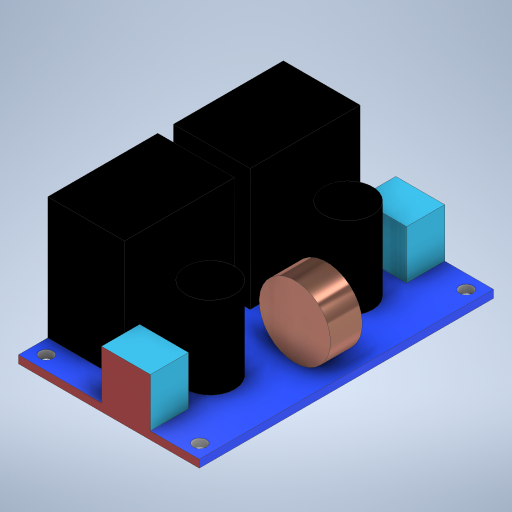
# Autodesk Inventor part: ConversosDCDC
Saved by Autodesk Inventor 2024 (Build 280153000, 153)
## iProperties
Created: 2024-05-29
Part Number: ConversosDCDC
Material: Genérico
Document SubType Name: Modeling
Designer: alexa
Density: 1 g/cm^3
Appearance: Valor por defecto
Author: alexa
Autodesk Inventor part; units mm, degrees
ref_plane "YZ Plane" through (0, 0, 0) normal (1, 0, 0) x (0, 1, 0)
sketch "Sketch1" plane through (0, 0, 0) normal (0, 1, 0) x (-1, 0, 0)
  line L0 (-18.5, 30.1) -> (18.5, 30.1)
  line L1 (18.5, 30.1) -> (18.5, -30.1)
  line L2 (18.5, -30.1) -> (-18.5, -30.1)
  line L3 (-18.5, -30.1) -> (-18.5, 30.1)
  line L4 (-18.5, 30.1) -> (18.5, -30.1) construction
  line L5 (18.5, 30.1) -> (-18.5, -30.1) construction
  point P0 (0, 0)
  dimension "d0" = 37
  dimension "d1" = 60.2
  constraints: 12 end point, 2 midpoint, 2 parallel, 1 horizontal, 1 perpendicular
  measures "d0" distance of L1.end L2.end
  measures "d1" distance of L0.end L1.end
extrude "Extrusion1" add sketch "Sketch1" along normal blind 1.6
sketch "Sketch2" plane through (0, 1.6, 0) normal (0, 1, 0) x (1, 0, 0)
  line L0 (-18.5, -30.1) -> (18.5, -30.1) projected
  line L1 (18.5, -30.1) -> (8.5, -30.1)
  line L2 (8.5, -30.1) -> (-1.5, -30.1)
  line L3 (-1.5, -30.1) -> (-1.5, -22.3)
  line L4 (-1.5, -22.3) -> (8.5, -22.3)
  line L5 (8.5, -22.3) -> (8.5, -30.1)
  point P0 (0, 0)
  point P1 (-1.5, -30.1)
  dimension "d4" = 10
  dimension "d5" = 10
  dimension "d6" = 7.8
  constraints: 10 end point, 2 parallel, 1 horizontal, 1 perpendicular, 1 point on line
  measures "d4" distance of L0.end L1.end
  measures "d5" distance of L3.end L4.end
  measures "d6" distance of L2.end L3.end
extrude "Extrusion2" add sketch "Sketch2" along normal blind 10
sketch "Sketch3" plane through (0, 1.6, 0) normal (0, 1, 0) x (1, 0, 0)
  line L0 (-18.5, -30.1) -> (18.5, -30.1) projected
  line L1 (18.5, -30.1) -> (4.75, -30.1)
  line L2 (4.75, -30.1) -> (4.75, -14.1)
  circle A0 centre (4.75, -14.1) radius 5
  point P0 (0, 0)
  dimension "d9" = 13.75
  dimension "d10" = 16
  dimension "d11" = 10
  constraints: 4 end point, 1 centre point, 1 coincident, 1 perpendicular, 1 point on line
  measures "d9" distance of L0.end L1.end
  measures "d10" distance of L1.end L2.end
  measures "d11" diameter of A0
extrude "Extrusion3" add sketch "Sketch3" along normal blind 16.8
sketch "Sketch4" plane through (0, 1.6, 0) normal (0, 1, 0) x (1, 0, 0)
  line L0 (-18.5, -30.1) -> (-1.5, -30.1) projected
  line L1 (-18.5, -30.1) -> (-18.5, -24.1)
  line L2 (-18.5, 30.1) -> (-18.5, -30.1) projected
  line L3 (-18.5, -24.1) -> (-2.8, -24.1)
  line L4 (-2.8, -24.1) -> (-2.8, -1.6)
  line L5 (-2.8, -1.6) -> (-18.5, -1.6)
  line L6 (-18.5, -1.6) -> (-18.5, -24.1)
  point P0 (0, 0)
  dimension "d14" = 6
  dimension "d15" = 15.7
  dimension "d16" = 22.5
  constraints: 10 end point, 2 perpendicular, 2 point on line, 1 collinear, 1 horizontal
  measures "d14" distance of L0.start L1.end
  measures "d15" distance of L1.end L3.end
  measures "d16" distance of L3.end L4.end
extrude "Extrusion4" add sketch "Sketch4" along normal blind 25
ref_plane "Work Plane1" through (18.5, 0, 0) normal (0, 0, -1) x (-1, 0, 0)
sketch "Sketch6" plane through (18.5, 0, 0) normal (0, 0, -1) x (-1, 0, 0)
  line L0 (0, 1.6) -> (0, 8.9)
  line L1 (0, 8.9) -> (7.3, 8.9)
  circle A0 centre (7.3, 8.9) radius 7.3
  point P0 (18.5, 0)
  dimension "d25" = 7.3
  dimension "d26" = 7.3
  dimension "d27" = 14.6
  constraints: 4 end point, 1 centre point, 1 coincident, 1 perpendicular, 1 vertical
  measures "d25" distance of L0.start L0.end
  measures "d26" distance of L0.end L1.end
  measures "d27" diameter of A0
extrude "Extrusion6" add sketch "Sketch6" against normal blind 3.25
mirror "Mirror2" about plane through (18.5, 0, 0) normal (0, 0, -1) of "Extrusion4", "Extrusion2", "Extrusion3", "Extrusion6"
sketch "Sketch7" plane through (0, 1.6, 0) normal (0, 1, 0) x (1, 0, 0)
  circle A0 centre (-15.65, 27.25) radius 1.35
  line L0 (-18.5, 30.1) -> (-18.5, 24.1) projected
  point P0 (0, 0)
  dimension "d32" = 2.7
  dimension "d36" = 2.85
  dimension "d37" = 2.85
  constraints: 1 centre point
  measures "d32" diameter of A0
  measures "d36" distance from line of L0 A0.centre
  measures "d37" horizontal distance of L0.start A0.centre
extrude "Extrusion7" cut sketch "Sketch7" against normal blind 3.25
ref_plane "Work Plane2" through (0.05, 0, 30.1) normal (1, 0, 0) x (0, 0, -1)
mirror "Mirror3" about plane through (0.05, 0, 30.1) normal (1, 0, 0) of "Extrusion7"
mirror "Mirror4" about plane through (18.5, 0, 0) normal (0, 0, -1) of "Extrusion7", "Mirror3"
body "Solid1"
